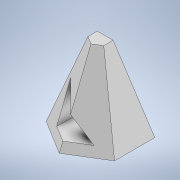
# Autodesk Inventor part: 1_1
Saved by Autodesk Inventor 2020.1 (Build 241239000, 239)
## iProperties
Created: 2022-02-16
Part Number: 1_1
Material: Типовые
Document SubType Name: Modeling
Designer: User
Density: 1 g/cm^3
Appearance: По умолчанию
Author: User
Autodesk Inventor part; units mm, degrees
sketch "Эскиз1" plane through (0, 0, 0) normal (0, 0, 1) x (1, 0, 0)
  line L0 (-53.4198, 62.894) -> (24.5802, 62.894)
  line L1 (24.5802, 62.894) -> (24.5802, -27.106)
  line L2 (24.5802, -27.106) -> (-53.4198, -27.106)
  line L3 (-53.4198, -27.106) -> (-53.4198, 62.894)
  line L4 (7.5802, -17.106) -> (-32.4198, -17.106)
  line L5 (-32.4198, -17.106) -> (-32.4198, 22.894)
  line L6 (-32.4198, 22.894) -> (7.5802, -17.106)
  point P0 (0, 0)
  point P1 (-14.4198, -27.106)
  point P2 (-14.4198, -17.106)
  dimension "d0" = 78
  dimension "d1" = 90
  dimension "d4" = 18
  dimension "d5" = 0
  dimension "d6" = 40
  dimension "d7" = 40
  dimension "d8" = 10
  constraints: 14 end point, 2 horizontal, 2 parallel, 2 perpendicular, 1 midpoint, 1 point on line
  measures "d0" distance of L1.end L2.end
  measures "d1" distance of L0.end L1.end
  measures "d4" distance of L4.end point (-14.42, -17.106)
  measures "d5" horizontal distance of point (-14.42, -27.106) point (-14.42, -17.106)
  measures "d6" distance of L4.start L4.end
  measures "d7" distance of L4.end L5.end
  measures "d8" distance from line of L2 L4.end
extrude "Выдавливание1" add sketch "Эскиз1" along normal blind 70
sketch "Эскиз3" plane through (-53.4198, 62.894, 0) normal (0, 1, 0) x (1, 0, 0)
  line L0 (78, -70) -> (0, -70) projected
  line L1 (39, -70) -> (78, -46)
  line L2 (78, 0) -> (78, -70) projected
  line L3 (78, 0) -> (0, 0) projected
  line L4 (39, -70) -> (0, -46)
  line L5 (0, 0) -> (0, -70) projected
  line L6 (0, -46) -> (0, 0)
  line L7 (0, 0) -> (78, 0)
  line L8 (78, 0) -> (78, -46)
  point P0 (53.4198, 0)
  dimension "d14" = 46
  constraints: 10 end point, 2 point on line, 1 horizontal, 1 midpoint, 1 perpendicular, 1 vertical
  measures "d14" distance from line of L3 L1.end
extrude "Выдавливание2" cut sketch "Эскиз3" against normal blind 1000 contours L4 L5 L3 L2 L1 keep common part
sketch "Эскиз4" plane through (-53.4198, 62.894, 0) normal (0, 1, 0) x (1, 0, 0)
  line L0 (78, 0) -> (0, 0) projected
  line L1 (0, 0) -> (78, 0)
  line L2 (0, 0) -> (0, -46) projected
  line L3 (0, -23) -> (78, -23)
  line L4 (78, 0) -> (78, -46) projected
  line L5 (39, -23) -> (78, 0)
  line L6 (78, -46) -> (39, -70) projected
  line L7 (39, -23) -> (78, -46)
  line L8 (39, -23) -> (0, -46)
  line L9 (39, -23) -> (0, 0)
  line L10 (30, -17.6923) -> (48, -17.6923)
  line L11 (48, -17.6923) -> (48, -28.3077)
  line L12 (48, -28.3077) -> (30, -28.3077)
  line L13 (30, -28.3077) -> (30, -17.6923)
  line L14 (39, -70) -> (61, -56.4615) projected
  line L15 (39, -23) -> (39, -70)
  line L16 (48, -28.3077) -> (39, -33.8468)
  line L17 (39, -33.8468) -> (30, -28.3077)
  point P0 (53.4198, 0)
  point P1 (39, -17.6923)
  point P2 (30, -23)
  dimension "d17" = 23
  dimension "d18" = 18
  dimension "d19" = 0
  dimension "d20" = 62.137
  dimension "d21" = 0
  dimension "d22" = 62.14
  constraints: 26 end point, 5 midpoint, 4 point on line, 3 horizontal, 2 parallel, 1 perpendicular, 1 vertical
  measures "d17" distance of L0.start L3.end
  measures "d18" distance of L10.start L10.end
  measures "d19" vertical distance of point (30, -23) L5.start
  measures "d20" angle of L6 L7
  measures "d21" distance of L11.end L16.start
  measures "d22" angle of L16 L7
ref_plane "РабПлоскость1" through (-53.4198, -27.106, 46) normal (-0.4959, 0.3237, 0.8058) x (0.8517, 0, 0.5241)
ref_plane "РабПлоскость2" through (24.5802, -27.106, 46) normal (-0.4959, -0.3237, -0.8058) x (-0.8517, 0, 0.5241)
ref_plane "РабПлоскость3" through (24.5802, -27.106, 0) normal (-0.9487, -0.3162, 0) x (0, 0, 1)
ref_plane "РабПлоскость4" through (-53.4198, -27.106, 0) normal (0, -0.1929, 0.9812) x (1, 0, 0)
ref_plane "РабПлоскость5" through (-53.4198, -27.106, 46) normal (0.9487, -0.3162, 0) x (0, 0, -1)
sketch "Эскиз5" plane through (24.5802, -27.106, 46) normal (-0.4959, -0.3237, -0.8058) x (-0.8517, 0, 0.5241)
  circle A0 centre (16.0933, 68.0296) radius 120.9619
  point P0 (-3.1746, 42.498)
  constraints: 1 centre point
extrude "Выдавливание3" cut sketch "Эскиз5" along normal blind 1000 keep common part
sketch "Эскиз6" plane through (-53.4198, -27.106, 46) normal (-0.4959, 0.3237, 0.8058) x (0.8517, 0, 0.5241)
  circle A0 centre (5.8398, 44.8642) radius 111.1599
  point P0 (21.3869, 47.3906)
  constraints: 1 centre point
extrude "Выдавливание4" cut sketch "Эскиз6" against normal blind 1000 keep common part
sketch "Эскиз7" plane through (24.5802, -27.106, 0) normal (-0.9487, -0.3162, 0) x (0, 0, 1)
  circle A0 centre (24.0277, 56.8574) radius 86.5432
  point P0 (0, 33.4879)
  constraints: 1 centre point
extrude "Выдавливание5" cut sketch "Эскиз7" along normal blind 1000 keep common part
sketch "Эскиз8" plane through (-53.4198, -27.106, 0) normal (0, -0.1929, 0.9812) x (1, 0, 0)
  circle A0 centre (24.124, 48.0247) radius 96.9769
  point P0 (53.4198, 26.5969)
  constraints: 1 centre point
extrude "Выдавливание6" cut sketch "Эскиз8" along normal blind 1000 keep common part
sketch "Эскиз9" plane through (-53.4198, -27.106, 46) normal (0.9487, -0.3162, 0) x (0, 0, -1)
  circle A0 centre (10.0162, 69.3054) radius 109.293
  point P0 (46, 42.6078)
  constraints: 1 centre point
extrude "Выдавливание7" cut sketch "Эскиз9" along normal blind 1000 keep common part
